spinner (Autodesk Fusion 360 design; units mm, degrees)
Autodesk Fusion 360 part; units mm, degrees
note: some values were not read from the file. Set by a fixed rule: which sketch regions a step uses.
sketch "Sketch1" plane through (0, 0, 0) normal (0, 1, 0) x (1, 0, 0)
  line L0 (0, -12.75) -> (0, -10.25)
  line L1 (0, -10.25) -> (-13, -10.25)
  line L2 (-13, -10.25) -> (-13, -4.4952)
  line L3 (-4, -5.075) -> (-4, -2.575)
  line L4 (-53, -2.575) -> (-53, -5)
  line L5 (-48, -4.7) -> (-48, -4.6)
  line L6 (-47.3, -3.9) -> (-45.7, -3.9)
  line L7 (-45, -4.6) -> (-45, -7.5)
  line L8 (-45, -7.5) -> (-42, -8.35)
  line L9 (-42, -8.35) -> (-17.5, -8.35)
  line L10 (-17.5, -8.35) -> (-13.5, -12.75)
  line L11 (-53, -5) -> (-52.0223, -5)
  line L12 (-49.15, -5) -> (-48.3, -5)
  arc A0 (-49.15, -5) -> (-52.0223, -5) centre (-50.5861, -6) ccw
  arc A1 (-47.3, -3.9) -> (-48, -4.6) centre (-47.3, -4.6) ccw
  arc A2 (-45, -4.6) -> (-45.7, -3.9) centre (-45.7, -4.6) ccw
  line L13 (-5.5, -5.075) -> (-4, -5.075)
  line L14 (-13.5, -12.75) -> (-12, -12.75)
  line L15 (-12, -12.75) -> (-12, -12.55)
  line L16 (-12, -12.55) -> (-2.5, -12.55)
  line L17 (-2.5, -12.55) -> (-2.5, -12.75)
  line L18 (-2.5, -12.75) -> (0, -12.75)
  circle A3 centre (-6.9856, -6) radius 1.75
  line L19 (-44.1316, -3.1) -> (-13.8684, -3.1)
  line L20 (-45.8554, -2.9503) -> (-48, -2.575)
  line L21 (-48, -2.575) -> (-53, -2.575)
  line L22 (-12.1446, -2.9503) -> (-10, -2.575)
  line L23 (-10, -2.575) -> (-4, -2.575)
  line L24 (-13, -4.4952) -> (-13, -4.4)
  line L25 (-12.5, -3.9) -> (-10.4711, -3.9)
  line L26 (-8.4711, -5.075) -> (-9.4711, -5.075)
  line L27 (-9.9711, -4.575) -> (-9.9711, -4.4)
  arc A4 (-12.5, -3.9) -> (-13, -4.4) centre (-12.5, -4.4) ccw
  arc A5 (-9.9711, -4.4) -> (-10.4711, -3.9) centre (-10.4711, -4.4) ccw
  arc A6 (-45.8554, -2.9503) -> (-44.1316, -3.1) centre (-44.1316, 6.9) ccw
  arc A7 (-13.8684, -3.1) -> (-12.1446, -2.9503) centre (-13.8684, 6.9) ccw
  line L28 (-48, -4.7) -> (-48.3, -5)
  line L29 (-9.4711, -5.075) -> (-9.9711, -4.575)
  point P0 (-48, -5)
  point P1 (-45, -3.1)
  point P2 (-13, -3.1)
  point P3 (-9.9711, -5.075)
  dimension "d2" = 2.5
  dimension "d5" = 2.5
  dimension "d6" = 13
  dimension "d8" = 53
  dimension "d10" = 5
  dimension "d12" = 5
  dimension "d14" = 8.35
  dimension "d15" = 7.5
  dimension "d17" = 3
  dimension "d19" = 3.5
  dimension "d21" = 0.7
  dimension "d39" = 0.7
  dimension "d40" = 1.15
  dimension "d41" = 6
  dimension "d42" = 8
  dimension "d43" = 0.7
  dimension "d44" = 17.5
  dimension "d45" = 13.5
  dimension "d46" = 9.5
  dimension "d47" = 2.5
  dimension "d48" = 0.2
  dimension "d49" = 12.75
  dimension "d50" = 3.5
  dimension "d52" = 6
  dimension "d53" = 1.5
  dimension "d55" = 3.1
  dimension "d56" = 3
  dimension "d57" = 2.575
  dimension "d58" = 3
  dimension "d60" = 0.8
  dimension "d61" = 0.8
  dimension "d62" = 0.5
  dimension "d63" = 1.5
  dimension "d64" = 9
  dimension "d65" = 10
  dimension "d66" = 10
  dimension "d67" = 0.3
  dimension "d68" = 0.3
  dimension "d69" = 0.5
  dimension "d70" = 0.5
  constraint vertical L0
  constraint perpendicular L0 L1
  constraint perpendicular L1 L2
  constraint perpendicular L3 L9
  constraint coincident origin L0
  constraint tangent L5 A1
  constraint equal A1 A2
  constraint vertical L7
  constraint horizontal L11
  constraint horizontal L12
  constraint horizontal A1.centre A2.centre
  constraint vertical L5
  constraint coincident L4.end L11.start
  constraint collinear L11 L12
  constraint horizontal L14
  constraint perpendicular L14 L15
  constraint perpendicular L15 L16
  constraint perpendicular L16 L17
  constraint perpendicular L0 L18
  constraint collinear L14 L18
  constraint coincident L13.start A3
  constraint perpendicular L4 L19
  constraint horizontal L21
  constraint horizontal L23
  constraint collinear L21 L23
  constraint coincident L7 P1
  constraint coincident L2 P2
  constraint perpendicular L9 L24
  constraint perpendicular L24 L25
  constraint horizontal L13
  constraint horizontal L25
  constraint coincident A3 L26.start
  constraint parallel L9 L26
  constraint collinear L13 L26
  constraint vertical L27
  constraint tangent L24 A4
  constraint tangent L25 A4
  constraint tangent L25 A5
  constraint tangent L27 A5
  constraint equal A4 A5
  constraint coincident P1 L19
  constraint coincident P1 L20
  constraint tangent L19 A6
  constraint tangent L20 A6
  constraint coincident P2 L19
  constraint coincident P2 L22
  constraint tangent L19 A7
  constraint tangent L22 A7
  constraint coincident P0 L5
  constraint coincident P0 L12
  constraint coincident P3 L26
  constraint coincident P3 L27
  measures "d2" distance of L0.start L0.end
  measures "d5" distance of L3.start L3.end
  measures "d6" distance of L0 L2
  measures "d8" distance of origin L4
  measures "d10" distance of origin L11
  measures "d12" distance of L4.end P0
  measures "d14" distance of origin L9
  measures "d15" vertical distance of origin L7.end
  measures "d17" horizontal distance of L7.end L8.end
  measures "d19" diameter of A0
  measures "d21" radius of A1
  measures "d39" distance of L6 A1.centre
  measures "d40" distance of P0 L12.start
  measures "d41" vertical distance of origin A0.centre
  measures "d42" distance of L4 L7
  measures "d43" horizontal distance of L7.start A2.centre
  measures "d44" distance of L0 L9.end
  measures "d45" distance of L0.start L10.end
  measures "d46" distance of L15.end L16.end
  measures "d47" distance of L0.start L17.end
  measures "d48" distance of L16.end L17.end
  measures "d49" distance of origin L14
  measures "d50" diameter of A3
  measures "d52" vertical distance of origin A3.centre
  measures "d53" distance of L3.start L13.start
  measures "d55" distance of origin L19
  measures "d56" horizontal distance of P2 L22.end
  measures "d57" distance of origin L23
  measures "d58" horizontal distance of P1 L20.end
  measures "d60" distance of L6 L19
  measures "d61" distance of P2 L25
  measures "d62" radius of A4
  measures "d63" distance of L26.start P3
  measures "d64" distance of L2 L3
  measures "d65" radius of A6
  measures "d66" radius of A7
  measures "d67" distance of P0 L5.start
  measures "d68" distance of P0 L12.end
  measures "d69" distance of P3 L26.end
  measures "d70" distance of P3 L27.start
revolve "Revolve1" add sketch "Sketch1" angle 360 about axis through (1.75, 0, 0) along (1, 0, 0) contours L0 L1 L2 L3 L4 L5 L6 L7 L8 L9 L10 L11 L12 A0 A1 A2 L13 L14 L15 L16 L17 L18 A3 L19 L20 L21 L22 L23 L24 L25 L26 L27 A4 A5 A6 A7 L28 L29
sketch "Sketch2" plane through (-53, 0, 0) normal (-1, 0, 0) x (0, -1, 0)
  circle A0 centre (0, 0) radius 5
  line L0 (-1, 6) -> (1, 6)
  line L1 (1, 6) -> (1, 0)
  line L2 (1, 0) -> (-1, 0)
  line L3 (-1, 0) -> (-1, 6)
  circle A1 centre (0, 0) radius 2.575
  dimension "d25" = 2
  dimension "d26" = 6
  constraint horizontal L0
  constraint vertical L1
  constraint horizontal L2
  constraint vertical L3
  constraint midpoint A0.centre L2
  measures "d25" distance of L0.start L0.end
  measures "d26" distance of L0.start L2.end
extrude "Extrude1" cut sketch "Sketch2" against normal blind 8 contours A0 L1 L3 A1 picked at (0, 4.1842)
pattern_circular "C-Pattern1" count 3 over 360 about axis through (1.75, 0, 0) along (1, 0, 0) of "Extrude1"
sketch "Sketch3" plane through (0, 0, 0) normal (1, 0, 0) x (0, 1, 0)
  line L0 (-1, 0) -> (1, 0)
  line L1 (1, 0) -> (1, 6)
  line L2 (1, 6) -> (-1, 6)
  line L3 (-1, 6) -> (-1, 0)
  dimension "d31" = 2
  dimension "d32" = 6
  constraint horizontal L0
  constraint vertical L1
  constraint horizontal L2
  constraint vertical L3
  constraint midpoint origin L0
  measures "d31" distance of L1.end L2.end
  measures "d32" distance of L0.start L2.end
extrude "Extrude2" cut sketch "Sketch3" against normal up to surface (13 mm away)
pattern_circular "C-Pattern2" count 3 over 360 about axis through (1.75, 0, 0) along (1, 0, 0) of "Extrude2"
equation "d14 = 16.7 mm / 2"
equation "d15 = ( 15 / 2 ) * 1 mm"
equation "d39 = d21"
equation "d41 = ( 12 / 2 ) * 1 mm"
equation "d43 = d21"
equation "d49 = ( 25.5 / 2 ) * 1 mm"
equation "d68 = d67"
equation "d70 = d69"
